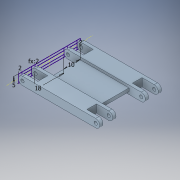
# Autodesk Inventor part: Bottom-Lip
Saved by Autodesk Inventor 2018.3 (Build 223284000, 284)
## iProperties
Created: 2018-05-17
Part Number: Bottom-Lip
Material: Generisch
Document SubType Name: Modeling
Designer: JochenAlt
Density: 1 g/cm^3
Appearance: Vorgabe
Author: JochenAlt
Autodesk Inventor part; units mm, degrees
ref_plane "YZ Plane" through (0, 0, 0) normal (1, 0, 0) x (0, 1, 0)
ref_plane "XZ Plane" through (0, 0, 0) normal (0, 1, 0) x (-1, 0, 0)
ref_plane "XY Plane" through (0, 0, 0) normal (0, 0, 1) x (1, 0, 0)
sketch "Skizze1" plane through (0, 0, 0) normal (1, 0, 0) x (0, 1, 0)
  line L0 (0, 3.5) -> (0, -3.5) construction
  line L1 (-26.6, 0) -> (26.6, 0) construction
  line L2 (19, 2.5) -> (9, 2.5)
  line L3 (9, 2.5) -> (9, -2.5)
  line L4 (9, -2.5) -> (19, -2.5)
  line L5 (19, -2.5) -> (19, 2.5)
  line L6 (-9, 2.5) -> (-19, 2.5)
  line L7 (-19, 2.5) -> (-19, -2.5)
  line L8 (-19, -2.5) -> (-9, -2.5)
  line L9 (-9, -2.5) -> (-9, 2.5)
  line L10 (9, 2.5) -> (-9, 2.5)
  line L11 (9, -2.5) -> (-9, -2.5)
  line L12 (19, 1) -> (-19, 1)
  line L13 (-19, 1) -> (-19, -1)
  line L14 (-19, -1) -> (19, -1)
  line L15 (19, -1) -> (19, 1)
  line L16 (-17, 2.5) -> (-17, -2.5)
  line L17 (-11, 2.5) -> (-11, -2.5)
  line L18 (11, 2.5) -> (11, -2.5)
  line L19 (17, 2.5) -> (17, -2.5)
  dimension "d0" = 10
  dimension "d1" = 18
  dimension "d6" = 2
  dimension "d14" = 5
  dimension "d20" = 2
  dimension "d21" = 2
  constraints: 36 end point, 10 point on line, 6 parallel, 5 perpendicular, 4 horizontal, 3 vertical, 1 collinear, 5 other
  measures "d0" distance of L3.end L4.end
  measures "d1" distance between parallel lines of L9 L3
  measures "d6" distance of L14.end L12.start
  measures "d14" distance of L6.end L7.end
  measures "d20" distance between parallel lines of L16 L7
  measures "d21" distance between parallel lines of L9 L17
extrude "Extrusion3" add sketch "Skizze1" along normal blind 50 contours L5 L14 L19 L12 | L19 L14 L18 L12 | L18 L14 L3 L12 | L3 L14 L9 L12 | L9 L14 L17 L12 | L17 L14 L16 L12 | L16 L14 L7 L12
extrude "Extrusion4" add sketch "Skizze1" along normal blind 50 contours L5 L12 L19 L2 | L19 L12 L18 L2 | L5 L14 L19 L12 | L18 L12 L3 L2 | L19 L14 L18 L12 | L5 L4 L19 L14 | L18 L14 L3 L12 | L19 L4 L18 L14 | L9 L12 L17 L6 | L18 L4 L3 L14 | L9 L14 L17 L12 | L17 L12 L16 L6 | L9 L8 L17 L14 | L17 L14 L16 L12 | L16 L12 L7 L6 | L17 L8 L16 L14 | L16 L14 L7 L12 | L16 L8 L7 L14
extrude "Extrusion5" cut sketch "Skizze1" along normal blind 10 contours L19 L12 L18 L2 | L19 L14 L18 L12 | L3 L12 L9 L10 | L19 L4 L18 L14 | L3 L14 L9 L12 | L3 L11 L9 L14 | L17 L12 L16 L6 | L17 L14 L16 L12 | L17 L8 L16 L14
fillet "Rundung2" radius 2.5 8 edges at (0, -10, -2.5) (0, -18, -2.5) (0, 18, -2.5) (0, 10, -2.5) (0, -18, 2.5) (0, -10, 2.5) (0, 10, 2.5) (0, 18, 2.5)
extrude "Extrusion7" cut sketch "Skizze1" against normal blind 10 from surface at 50 contours L19 L12 L18 L2 | L19 L14 L18 L12 | L3 L12 L9 L10 | L19 L4 L18 L14 | L3 L14 L9 L12 | L3 L11 L9 L14 | L17 L12 L16 L6 | L17 L14 L16 L12 | L17 L8 L16 L14
fillet "Rundung4" radius 2.5 8 edges at (50, -10, 2.5) (50, -18, 2.5) (50, -18, -2.5) (50, 10, 2.5) (50, 18, 2.5) (50, 18, -2.5) (50, 10, -2.5) (50, -10, -2.5)
sketch "Skizze2" plane through (50, 19, 1) normal (0, 1, 0) x (1, 0, 0)
  circle A0 centre (-47.5, 1) radius 1
  arc A1 (-47.5, 3.5) -> (-47.5, -1.5) centre (-47.5, 1) ccw projected
  circle A2 centre (-2.5, 1) radius 1
  arc A3 (-2.5, -1.5) -> (-2.5, 3.5) centre (-2.5, 1) ccw projected
  point P0 (-50, 1)
  dimension "d16" = 2
  constraints: 2 centre point, 2 concentric, 1 equal radius
  measures "d16" diameter of A0
extrude "Extrusion6" cut sketch "Skizze2" against normal through all
equation "\"d21\" = d20"
equation "\"d15\" = 0.5 * d14"
equation "\"d24\" = 0.5 * d14"
